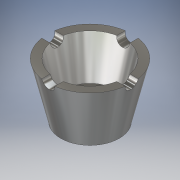
# Autodesk Inventor part: Screw Jack Cup
Saved by Autodesk Inventor 2018 (Build 220112000, 112)
## iProperties
Created: 2019-08-31
Part Number: Screw Jack Cup
Material: Generic
Document SubType Name: Modeling
Designer: HP
Density: 1 g/cm^3
Appearance: Chrome - Polished
Author: HP
Autodesk Inventor part; units mm, degrees
ref_plane "YZ Plane" through (0, 0, 0) normal (1, 0, 0) x (0, 1, 0)
ref_plane "XZ Plane" through (0, 0, 0) normal (0, 1, 0) x (-1, 0, 0)
ref_plane "XY Plane" through (0, 0, 0) normal (0, 0, 1) x (1, 0, 0)
sketch "Sketch1" plane through (0, 0, 0) normal (0, 0, 1) x (1, 0, 0)
  line L0 (11, 0) -> (22.5, 0)
  line L1 (11, 0) -> (11, 12)
  line L2 (11, 12) -> (19, 12)
  line L3 (32.5, 42) -> (22.5, 0)
  line L4 (19, 12) -> (26.1429, 42)
  line L5 (26.1429, 42) -> (32.5, 42)
  line L6 (0, -8.4) -> (0, 50.4) projected
  point P0 (0, 0)
  dimension "d0" = 11.5
  dimension "d1" = 11
  dimension "d2" = 22.5
  dimension "d3" = 12
  dimension "d4" = 19
  dimension "d5" = 8
  dimension "d7" = 6.1843
  dimension "d8" = 32.5
  dimension "d9" = 42
  constraints: 12 end point, 3 horizontal, 1 parallel, 1 point on line, 1 vertical
  measures "d0" distance of L0.start L0.end
  measures "d1" distance of L0.start point (0, 0)
  measures "d2" distance of L0.end point (0, 0)
  measures "d3" distance of L0.start L1.end
  measures "d4" horizontal distance of L2.end point (0, 0)
  measures "d5" distance of L1.end L2.end
  measures "d7" distance between parallel lines of L3 L4
  measures "d8" horizontal distance of L3.start point (0, 0)
  measures "d9" distance from line of L0 L3.start
revolve "Revolution1" add sketch "Sketch1" angle 360 about axis through (0, -10, 0) along (0, 1, 0)
sketch "Sketch2" plane through (0, 0, 0) normal (0, 0, 1) x (1, 0, 0)
  line L0 (-32.5, 42) -> (32.5, 42) projected
  circle A0 centre (0, 42) radius 5
  point P0 (0, 0)
  dimension "d11" = 10
  constraints: 1 centre point, 1 midpoint
  measures "d11" diameter of A0
extrude "Extrusion1" cut sketch "Sketch2" along normal through all both and the other way through all
sketch "Sketch3" plane through (0, 0, 0) normal (1, 0, 0) x (0, 1, 0)
  line L0 (42, 25.6603) -> (42, -25.6603) projected
  circle A0 centre (42, 0) radius 5
  point P0 (0, 0)
  dimension "d14" = 10
  constraints: 1 centre point, 1 midpoint
  measures "d14" diameter of A0
extrude "Extrusion2" cut sketch "Sketch3" along normal through all both and the other way through all
body "Solid1"
